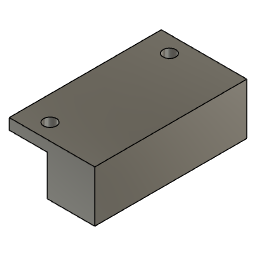
Cubesat 3u v11 (Autodesk Fusion 360 archive; units mm, degrees)
design "датчик света"
Autodesk Fusion 360 part; units mm, degrees
sketch "Sketch1" plane through (0, 0, 0) normal (0, 0, 1) x (1, 0, 0)
  line L0 (0, 35) -> (18, 35)
  line L1 (18, 35) -> (18, 3)
  line L2 (18, 3) -> (0, 3)
  line L3 (0, 3) -> (0, 35)
  line L4 (8, 19.5) -> (10, 19.5)
  line L5 (10, 19.5) -> (10, 18.5)
  line L6 (10, 18.5) -> (8, 18.5)
  line L7 (8, 19.5) -> (8, 18.5)
  circle A0 centre (5.1528, 6.4363) radius 1.35
  circle A1 centre (5.1528, 31.5637) radius 1.35
  line L8 (8, 25) -> (8, 35)
  line L9 (8, 25) -> (0, 25)
  line L10 (8, 13) -> (0, 13)
  line L11 (8, 13) -> (8, 3)
  dimension "d12" = 2.7
  constraint horizontal L0
  constraint vertical L1
  constraint horizontal L2
  constraint vertical L3
  constraint perpendicular L6 L7
  constraint coincident L0 L8.end
  constraint perpendicular L0 L8
  constraint coincident L3 L9.end
  constraint perpendicular L3 L9
  measures "d12" diameter of A0
extrude "Extrude1" add sketch "Sketch1" against normal blind 8.5 contours L0 L1 L2 L3 L8 L9 L10 L11 | L4 L5 L6 L7
extrude "Extrude2" add sketch "Sketch1" along normal blind 2.3
extrude "Extrude3" add 1 faces at (8.6667, 19.1667, 0) along direction (0, 0, 1) blind 2.3

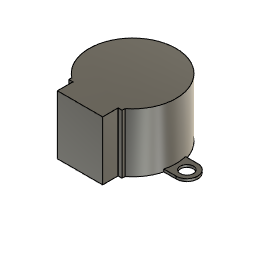
design "мотор"
Autodesk Fusion 360 part; units mm, degrees
sketch "Sketch1" plane through (0, 0, 0) normal (0, 0, 1) x (1, 0, 0)
  circle A0 centre (0, 0) radius 14
  circle A1 centre (0, 8) radius 4.5
  circle A2 centre (0, 8) radius 2.5
  line L0 (-2.5, 9.5) -> (-2.5, 6.5)
  line L1 (-2.5, 6.5) -> (2.5, 6.5)
  line L2 (2.5, 6.5) -> (2.5, 9.5)
  line L3 (-2.5, 9.5) -> (2.5, 9.5)
  line L4 (0, 0) -> (-17.5054, 0) construction
  line L5 (0, 0) -> (17.5, 0) construction
  circle A3 centre (-17.5054, 0) radius 2.1
  circle A4 centre (17.5, 0) radius 2.1
  arc A5 (-17.5054, 3.5) -> (-17.5054, -3.5) centre (-17.5054, 0) ccw
  line L6 (-17.5054, 3.5) -> (-13.5554, 3.5)
  line L7 (-17.5054, -3.5) -> (-13.5554, -3.5)
  line L8 (17.5054, 3.5) -> (13.5554, 3.5)
  arc A6 (17.5054, -3.5) -> (17.5054, 3.5) centre (17.5054, 0) ccw
  line L9 (17.5054, -3.5) -> (13.5554, -3.5)
  line L10 (0, 0) -> (0, -12) construction
  line L11 (0, 0) -> (0, -17) construction
  line L12 (0, -17) -> (7.3, -17)
  line L13 (0, -17) -> (-7.3, -17)
  line L14 (-7.3, -17) -> (-7.3, -11.9461)
  line L15 (7.3, -17) -> (7.3, -11.946)
  line L16 (0, -12) -> (8.6, -12)
  line L17 (8.6, -12) -> (-8.6, -12)
  line L18 (8.6, -12) -> (8.6, -11.0472)
  line L19 (-8.6, -12) -> (-8.6, -11.0472)
  dimension "d1" = 28
  dimension "d12" = 4.2
  constraint coincident A0.centre L4.start
  constraint concentric A1 A2
  constraint perpendicular L0 L1
  constraint perpendicular L1 L2
  constraint perpendicular L0 L3
  constraint parallel L3 L4
  constraint parallel L4 L5
  constraint coincident L4.end A3.centre
  constraint coincident L5.end A4.centre
  constraint coincident A0 L6.end
  constraint tangent A5 L6
  constraint coincident A0 L7.end
  constraint tangent A5 L7
  constraint perpendicular L5 L10
  constraint perpendicular L5 L11
  constraint perpendicular L11 L12
  constraint perpendicular L11 L13
  constraint coincident A0 L14.end
  constraint perpendicular L12 L15
  constraint perpendicular L15 L16
  constraint perpendicular L14 L17
  constraint coincident A0 L18.end
  constraint perpendicular L17 L18
  constraint coincident A0 L19.end
  constraint perpendicular L17 L19
  measures "d1" diameter of A0
  measures "d12" diameter of A4
extrude "Extrude1" add sketch "Sketch1" along normal blind 19 contours A0 L16 L17 | A0 L15 L16 L17 L18 | A0 L14 L17 L19 | A0 L12 L13 L14 L15 L16 L17 | A0 L16 L17 | A1 | A2 L1 L3 | A2 L1 L2 | A2 L2 L3 | A2 L3 | A2 L1 | A2 L0 L3 | A2 L0 L1 makes body 1
extrude "Extrude2" add sketch "Sketch1" along normal blind 0.8 separate body contours A0 L8 A6 L9 | A0 A5 L6 L7 makes body 2 at (-15.8388, 2.9396, 0) makes body 3 at (15.837, 2.9396, 0)
extrude "Extrude3" add sketch "Sketch1" against normal blind 2 separate body contours A1 | A2 L1 L3 | A2 L1 L2 | A2 L2 L3 | A2 L3 | A2 L1 | A2 L0 L3 | A2 L0 L1 makes body 4
extrude "Extrude4" cut sketch "Sketch1" against normal blind 4 contours A2 L1 L3 | A2 L3 | A2 L1 bodies 4
extrude "Extrude5" add sketch "Sketch1" against normal blind 4 separate body contours A2 L1 L3 | A2 L3 | A2 L1 makes body 5
sketch "Sketch2" plane through (0, 0, -4) normal (0, 0, -1) x (1, 0, 0)
  circle A0 centre (0, -8) radius 2.5
  line L0 (0, -8) -> (0, -6.5)
  line L1 (2, -9.5) -> (-2, -9.5)
  line L2 (2, -9.5) -> (1.8, -9.5)
  line L3 (2, -6.5) -> (-2, -6.5)
  constraint coincident A0.centre L0.start
  constraint vertical L0
  constraint coincident A0 L1.start
  constraint coincident A0 L1.end
  constraint coincident L1 L2.end
  constraint parallel L1 L2
  constraint coincident A0 L3.start
  constraint coincident A0 L3.end
extrude "Extrude6" add sketch "Sketch2" along normal blind 6 contours A0 L1 L2 L3 bodies 5
copy_body "CopyPasteBodies1" bodies 2 1 3 4 5 makes body 6 makes body 7 makes body 8 makes body 9 makes body 10
copy_body "CopyPasteBodies2" bodies 1 7 2 6 5 10 4 9 3 8 makes body 11 makes body 12 makes body 13 makes body 14 makes body 15 makes body 16 makes body 17 makes body 18 makes body 19 makes body 20
hidden bodies 18
